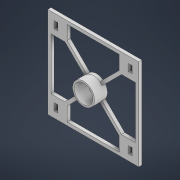
# Autodesk Inventor part: Joints_Remake_TestFit_V1
Saved by Autodesk Inventor 2022 (Build 260153000, 153)
## iProperties
Created: 2023-06-09
Part Number: Joints_Remake_TestFit_V1
Material: Generic
Document SubType Name: Modeling
Designer: Karl Spiteri
Density: 1 g/cm^3
Appearance: Default
Author: Karl Spiteri
Autodesk Inventor part; units mm, degrees
ref_plane "YZ Plane" through (0, 0, 0) normal (1, 0, 0) x (0, 1, 0)
ref_plane "XZ Plane" through (0, 0, 0) normal (0, 1, 0) x (-1, 0, 0)
ref_plane "XY Plane" through (0, 0, 0) normal (0, 0, 1) x (1, 0, 0)
sketch "Sketch1" plane through (0, 0, 0) normal (0, 0, 1) x (1, 0, 0)
  line L0 (0, 0) -> (-140, 0)
  line L1 (-140, 0) -> (-140, 140)
  line L2 (-140, 140) -> (0, 140)
  line L3 (0, 140) -> (0, 0)
  circle A0 centre (-70, 70) radius 14.35
  line L4 (-130, 124.4) -> (-130, 130)
  line L5 (-10, 124.4) -> (-10, 130)
  line L6 (-10, 15.6) -> (-10, 10)
  line L7 (-130, 15.6) -> (-130, 10)
  line L8 (-140, 140) -> (-110, 140)
  line L9 (-110.0005, 135.0005) -> (-110.0005, 113.536)
  line L10 (-113.536, 110) -> (-135, 110)
  line L11 (-140, 110) -> (-140, 140)
  line L12 (-140, 0) -> (-110, 0)
  line L13 (-109.9998, 5.0002) -> (-109.9998, 26.4642)
  line L14 (-113.536, 30) -> (-135, 30)
  line L15 (-140, 30) -> (-140, 0)
  line L16 (0, 0) -> (-30, 0)
  line L17 (-30, 5.0002) -> (-30, 26.464)
  line L18 (-26.4645, 30) -> (-5, 30)
  line L19 (0, 30) -> (0, 0)
  line L20 (0, 140) -> (-30, 140)
  line L21 (-30, 135.0005) -> (-30, 113.536)
  line L22 (-26.4638, 110.0002) -> (-5, 110.0002)
  line L23 (0, 110) -> (0, 140)
  line L24 (-110.0005, 113.536) -> (-80.0116, 83.5551)
  line L25 (-56.4494, 59.9849) -> (-26.4645, 30)
  line L26 (-113.536, 110) -> (-83.5508, 80.0148)
  line L27 (-59.9852, 56.4492) -> (-30, 26.464)
  line L28 (-113.536, 30) -> (-83.5508, 59.9852)
  line L29 (-59.9861, 83.5534) -> (-29.9997, 113.5363)
  line L30 (-109.9998, 26.4642) -> (-80.0148, 56.4492)
  line L31 (-56.4492, 80.0148) -> (-26.4638, 110.0002)
  line L32 (-135, 110) -> (-135, 30)
  line L33 (-140, 30) -> (-140, 110)
  line L34 (-5, 110.0002) -> (-5, 30)
  line L35 (0, 30) -> (0, 110)
  line L36 (-110, 140) -> (-30, 140)
  line L37 (-30, 135.0005) -> (-110.0005, 135.0005)
  line L38 (-30, 0) -> (-110, 0)
  line L39 (-109.9998, 5.0002) -> (-30, 5.0002)
  arc A1 (-83.5508, 80.0148) -> (-83.5508, 59.9852) centre (-70, 70) ccw
  arc A2 (-59.9861, 83.5534) -> (-80.0116, 83.5551) centre (-70, 70) ccw
  arc A3 (-80.0148, 56.4492) -> (-59.9852, 56.4492) centre (-70, 70) ccw
  arc A4 (-56.4494, 59.9849) -> (-56.4492, 80.0148) centre (-70, 70) ccw
  line L40 (-130, 130) -> (-124.4, 130)
  line L41 (-124.4, 130) -> (-124.4, 119.4)
  line L42 (-124.4, 119.4) -> (-130, 119.4)
  line L43 (-130, 119.4) -> (-130, 130)
  line L44 (-130, 10) -> (-124.4, 10)
  line L45 (-124.4, 10) -> (-124.4, 20.6)
  line L46 (-124.4, 20.6) -> (-130, 20.6)
  line L47 (-130, 20.6) -> (-130, 10)
  line L48 (-10, 10) -> (-15.6, 10)
  line L49 (-15.6, 10) -> (-15.6, 20.6)
  line L50 (-15.6, 20.6) -> (-10, 20.6)
  line L51 (-10, 20.6) -> (-10, 10)
  line L52 (-10, 130) -> (-15.6, 130)
  line L53 (-15.6, 130) -> (-15.6, 119.4)
  line L54 (-15.6, 119.4) -> (-10, 119.4)
  line L55 (-10, 119.4) -> (-10, 130)
  line L56 (-113.536, 30) -> (-109.9998, 26.4642)
  line L57 (-30, 26.464) -> (-26.4645, 30)
  line L58 (-30, 113.536) -> (-26.4638, 110.0002)
  line L59 (-110.0005, 113.536) -> (-113.536, 110)
  point P0 (-110, 113.5355)
  point P1 (-110, 26.464)
  point P2 (-26.464, 110)
  constraints: 120 end point, 22 parallel, 12 perpendicular, 11 horizontal, 8 point on circle, 5 centre point, 1 coincident, 1 point on line
extrude "Extrusion2" add sketch "Sketch1" along normal blind 5 contours L0 L1 L2 L3 | L24 A2 L29 L58 L31 A4 L25 L57 L27 A3 L30 L56 L28 A1 L26 L59
sketch "Sketch2" plane through (0, 0, 5) normal (0, 0, 1) x (1, 0, 0)
  circle A0 centre (-70, 70) radius 14.35 projected
  circle A1 centre (-70, 70) radius 16.85
  circle A2 centre (-70, 70) radius 14.35
  point P0 (0, 0)
  dimension "d59" = 33.7
  dimension "d60" = 28.7
  constraints: 2 centre point, 2 coincident
  measures "d59" diameter of A1
  measures "d60" diameter of A2
extrude "Extrusion3" add sketch "Sketch2" along normal blind 15
body "Solid2"
